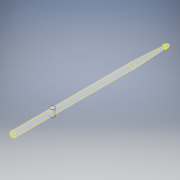
# Autodesk Inventor part: stickROCK
Saved by Autodesk Inventor 2019 (Build 230136000, 136)
## iProperties
Created: 2013-05-05
Part Number: stickROCK
Material: Generic
Description: SolidWorks IGES file using analytic representation for surfaces
Document SubType Name: Modeling
Designer: Lenovo
Density: 1 g/cm^3
Appearance: Default
Title: X:\Datoteke\Exp\CAD\drumsticks\ROCK\stickROCK.IGS
Author: Spitfire
Sending System: SolidWorks 2011
Preprocessor: SolidWorks 2011
Minimum Resolution: 0.0
Sending System Product ID: stickROCK
Receiving System Product ID: stickROCK
Sent Units: Inch
Translation Standard: IGES 5.3
Model Creation Time: 2013-05-05
Autodesk Inventor part; units mm, degrees
ref_plane "YZ Plane" through (0, 0, 0) normal (1, 0, 0) x (0, 1, 0)
ref_plane "XZ Plane" through (0, 0, 0) normal (0, 1, 0) x (-1, 0, 0)
ref_plane "XY Plane" through (0, 0, 0) normal (0, 0, 1) x (1, 0, 0)
surface "Composite1"
sketch "Sketch1" plane through (0, 0, 0) normal (0, 1, 0) x (-1, 0, 0)
  circle A0 centre (0, -111.125) radius 6.35
  point P0 (0, 0)
  constraints: 1 centre point
extrude "Extrusion1" add sketch "Sketch1" along normal blind 8.89 and the other way blind 8.89
sketch "Sketch2" plane through (0, -8.89, -111.125) normal (0, -1, 0) x (1, 0, 0)
  point P0 (0, 111.125)
  point P1 (-0.354, -0.8362)
hole "Hole1" at (-0.354, -8.89, -111.9612) direction (0, -1, 0) diameter 0.5 depth 0.5
body "Solid1"
body "Srf1"
